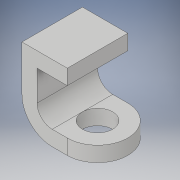
# Autodesk Inventor part: 40823233
Saved by Autodesk Inventor 2019 (Build 230136000, 136)
## iProperties
Created: 2021-01-08
Part Number: 40823233
Material: 一般
Document SubType Name: Modeling
Designer: user
Density: 1 g/cm^3
Appearance: 預設
Author: user
Autodesk Inventor part; units mm, degrees
ref_plane "YZ Plane" through (0, 0, 0) normal (1, 0, 0) x (0, 1, 0)
ref_plane "XZ Plane" through (0, 0, 0) normal (0, 1, 0) x (-1, 0, 0)
ref_plane "XY Plane" through (0, 0, 0) normal (0, 0, 1) x (1, 0, 0)
sketch "草圖1" plane through (0, 0, 0) normal (0, 0, 1) x (1, 0, 0)
  line L0 (20, 0) -> (40, 0)
  line L1 (30, 50) -> (0, 50)
  line L2 (0, 50) -> (0, 20)
  arc A0 (0, 20) -> (20, 0) centre (20, 20) ccw
  line L3 (30, 50) -> (30, 40)
  line L4 (30, 40) -> (10, 40)
  line L5 (10, 40) -> (10, 20)
  arc A1 (10, 20) -> (20, 10) centre (20, 20) ccw
  line L6 (40, 10) -> (20, 10)
  line L7 (40, 0) -> (50, 0)
  line L8 (50, 0) -> (50, 10)
  line L9 (50, 10) -> (40, 10)
  point P0 (0, 0)
  dimension "d0" = 30
  dimension "d1" = 10
  dimension "d9" = 10
  dimension "d10" = 20
  dimension "d11" = 20
  dimension "d17" = 10
  dimension "d18" = 10
  constraints: 20 end point, 4 perpendicular, 4 point on circle, 3 horizontal, 2 centre point, 1 coincident, 1 parallel, 1 tangent, 1 vertical
  measures "d0" distance of L1.end L1.start
  measures "d1" distance of L6.start L0.end
  measures "d9" distance of L1.start L3.end
  measures "d10" distance of L3.end L4.end
  measures "d11" distance of L4.end L5.end
  measures "d17" distance of L0.end L7.end
  measures "d18" distance of L7.end L8.end
extrude "擠出1" add sketch "草圖1" along normal blind 40
sketch "草圖2" plane through (20, 10, 0) normal (0, 1, 0) x (1, 0, 0)
  circle A0 centre (10, -20) radius 10
  point P0 (-20, 0)
  dimension "d14" = 20
  constraints: 1 centre point
  measures "d14" diameter of A0
extrude "擠出2" cut sketch "草圖2" against normal blind 40
sketch "草圖3" plane through (20, 10, 0) normal (0, 1, 0) x (1, 0, 0)
  line L0 (30, 0) -> (0, 0) projected
  line L1 (30, 0) -> (30, -40) projected
  line L2 (30, -40) -> (0, -40) projected
  arc A0 (10, -40) -> (10, 0) centre (10, -20) ccw
  line L3 (10, -40) -> (30, -40)
  line L4 (30, -20) -> (30, 0)
  point P0 (-20, 0)
  dimension "d20" = 40
  constraints: 4 end point, 3 point on circle, 2 collinear, 2 point on line, 1 centre point, 1 coincident, 1 midpoint
  measures "d20" diameter of A0
extrude "擠出3" cut sketch "草圖3" against normal blind 40
